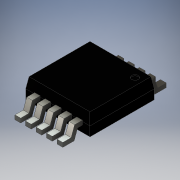
# Autodesk Inventor part: MAX17552
Saved by Autodesk Inventor 2016 (Build 200138000, 138)
## iProperties
Created: 2016-08-10
Part Number: MAX17552
Material: Generic
Document SubType Name: Modeling
Designer: jfixelle
Density: 1 g/cm^3
Appearance: Black
Author: jfixelle
Autodesk Inventor part; units mm, degrees
ref_plane "YZ Plane" through (0, 0, 0) normal (1, 0, 0) x (0, 1, 0)
ref_plane "XZ Plane" through (0, 0, 0) normal (0, 1, 0) x (-1, 0, 0)
sketch "Sketch1" plane through (0, 0, 0) normal (0, 1, 0) x (-1, 0, 0)
  line L0 (1.525, 1.525) -> (-1.525, 1.525)
  line L1 (-1.525, 1.525) -> (-1.525, -1.525)
  line L2 (-1.525, -1.525) -> (1.525, -1.525)
  line L3 (1.525, -1.525) -> (1.525, 1.525)
  point P0 (0, 0)
  dimension "d0" = 3.05
  dimension "d1" = 1.525
  dimension "d2" = 3.05
  dimension "d3" = 1.525
  constraints: 8 end point, 2 parallel, 1 horizontal, 1 perpendicular
  measures "d0" distance of L1.end L2.end
  measures "d1" distance from line of L3 point (0, 0)
  measures "d2" distance of L0.end L1.end
  measures "d3" distance from line of L2 point (0, 0)
extrude "Extrusion1" add sketch "Sketch1" along normal blind 0.95
chamfer "Chamfer1" distance 0.5 angle 9 1 edges at (0, 0.95, 1.525) measured on face at (-0.5083, 0.3167, 1.525)
chamfer "Chamfer2" distance 0.5 angle 9 1 edges at (1.525, 0.95, -0.0396) measured on face at (1.525, 0.6333, -0.5347)
chamfer "Chamfer3" distance 0.5 angle 9 1 edges at (-1.525, 0.95, -0.0396) measured on face at (-1.525, 0.6333, -0.5347)
chamfer "Chamfer4" distance 0.5 angle 9 1 edges at (0, 0.95, -1.525) measured on face at (0.4819, 0.6167, -1.525)
ref_plane "Work Plane1" through (1.027, 0, 1.525) normal (1, 0, 0) x (0, 0, -1)
sketch "Sketch2" plane through (1.027, 0, 1.525) normal (1, 0, 0) x (0, 0, -1)
  line L0 (3.0361, 0.5) -> (3.0361, 0.3)
  line L1 (3.0361, 0.3) -> (3.2761, 0.3)
  line L2 (3.2761, 0.3) -> (3.4387, -0.15)
  line L3 (3.4387, -0.15) -> (3.9761, -0.15)
  line L4 (3.9761, -0.15) -> (3.9761, 0.05)
  line L5 (3.9761, 0.05) -> (3.5802, 0.05)
  line L6 (3.5802, 0.05) -> (3.4176, 0.5)
  line L7 (3.4176, 0.5) -> (3.0361, 0.5)
  line L8 (3.05, 0) -> (3.05, 0.45) projected
  line L9 (0, 0) -> (3.05, 0) projected
  point P0 (1.525, 0)
  dimension "d20" = 0.2
  dimension "d21" = 0.2
  dimension "d22" = 0.7
  dimension "d23" = 0.94
  dimension "d24" = 0.65
  dimension "d25" = 0.15
  constraints: 16 end point, 3 parallel, 3 perpendicular, 1 vertical
  measures "d20" distance of L0.start L0.end
  measures "d21" distance of L3.end L4.end
  measures "d22" distance from line of L1.end L4
  measures "d23" distance between parallel lines of L4 L0
  measures "d24" distance between parallel lines of L3 L7
  measures "d25" distance between parallel lines of L9 L3
extrude "Extrusion2" add sketch "Sketch2" along normal mid plane 0.27
pattern_linear "Rectangular Pattern1" count 5 spacing 0.5 along (-1, 0, 0) of "Extrusion2"
mirror "Mirror1" about plane through (0, 0, 0) normal (0, 0, 1) of "Extrusion2", "Rectangular Pattern1"
sketch "Sketch3" plane through (0, 0.95, 0) normal (0, 1, 0) x (1, 0, 0)
  circle A0 centre (1.1025, 1.0346) radius 0.1629
  point P0 (0, 0)
  constraints: 1 centre point
extrude "Extrusion3" cut sketch "Sketch3" against normal blind 0.05
body "Solid1"
